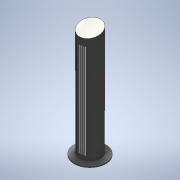
# Autodesk Inventor part: fan
Saved by Autodesk Inventor 2022 (Build 260153000, 153)
## iProperties
Created: 2023-01-12
Part Number: fan
Material: Generic
Document SubType Name: Modeling
Designer: mihir
Density: 1 g/cm^3
Appearance: Default
Author: mihir
Autodesk Inventor part; units mm, degrees
ref_plane "XY Plane" through (0, 0, 0) normal (0, 0, 1) x (1, 0, 0)
sketch "Sketch1" plane through (0, 0, 0) normal (0, 1, 0) x (-1, 0, 0)
  circle A0 centre (0, 0) radius 15
  dimension "d0" = 30
  constraints: 1 centre point, 1 coincident
  measures "d0" diameter of A0
ref_plane "Work Plane1" through (0, 1, 0) normal (0, 1, 0) x (-1, 0, 0)
sketch "Sketch2" plane through (0, 1, 0) normal (0, 1, 0) x (-1, 0, 0)
  circle A0 centre (0, 0) radius 15
  dimension "d2" = 30
  constraints: 1 centre point, 1 coincident
  measures "d2" diameter of A0
ref_plane "Work Plane2" through (0, 2, 0) normal (0, 1, 0) x (-1, 0, 0)
sketch "Sketch4" plane through (0, 2, 0) normal (0, 1, 0) x (-1, 0, 0)
  circle A0 centre (0, 0) radius 10
  dimension "d11" = 20
  constraints: 1 centre point, 1 coincident
  measures "d11" diameter of A0
loft "Loft2" add profiles "Sketch1", "Sketch2"
loft "Loft3" add profiles "Sketch4" section 1 edges at (15, 1, 0)
extrude "Extrusion1" add sketch "Sketch4" along normal blind 100
sketch "Sketch5" plane through (0, 0, 0) normal (0, 0, 1) x (1, 0, 0)
  line L0 (10, 102) -> (-10, 102) projected
  line L1 (-10, 102) -> (10, 102)
  line L2 (10, 102) -> (10, 107)
  line L3 (-10, 102) -> (-10, 102.5)
  line L4 (-10, 102.5) -> (10, 107)
  point P0 (0, 0)
  dimension "d22" = 5
  dimension "d23" = 0.5
  constraints: 8 end point, 1 collinear, 1 perpendicular, 1 vertical
  measures "d22" distance of L0.start L2.end
  measures "d23" distance of L0.end L3.end
extrude "Extrusion2" add sketch "Sketch5" along normal mid plane 20
fillet "Fillet1" radius 10 4 edges at (10, 104.5, 10) (10, 104.5, -10) (-10, 102.25, 10) (-10, 102.25, -10)
ref_plane "Work Plane3" through (-10, 0, 0) normal (1, 0, 0) x (0, 1, 0)
sketch "Sketch6" plane through (-10, 0, 0) normal (1, 0, 0) x (0, 1, 0)
  line L0 (96, -5) -> (6, -5)
  line L1 (6, -5) -> (6, 5)
  line L2 (6, 5) -> (96, 5)
  line L3 (96, 5) -> (96, -5)
  line L4 (0, -15) -> (0, 15) projected
  line L5 (0, -15) -> (1, -15)
  line L6 (0, -15) -> (1, -15) projected
  line L7 (1, 15) -> (1, -15) projected
  line L8 (96, -4) -> (6, -4)
  line L9 (6, -3.5) -> (96, -3.5)
  line L10 (96, -2.5) -> (6, -2.5)
  line L11 (6, -2) -> (96, -2)
  line L12 (96, -1) -> (6, -1)
  line L13 (6, -1) -> (96, -1)
  line L14 (96, -0.5) -> (6, -0.5)
  line L15 (6, 0.5) -> (96, 0.5)
  line L16 (96, 1) -> (6, 1)
  line L17 (96, 2) -> (6, 2)
  line L18 (96, 5) -> (6, 5)
  line L19 (96, 2.5) -> (6, 2.5)
  line L20 (2, 10) -> (104.75, 10) projected
  line L21 (6, 3.5) -> (96, 3.5)
  line L22 (96, 4) -> (6, 4)
  line L23 (6, 4) -> (96, 4)
  point P0 (0, 0)
  point P1 (6, 2.5)
  point P2 (6, 1)
  dimension "d28" = 90
  dimension "d29" = 10
  dimension "d30" = 10
  dimension "d31" = 5
  dimension "d34" = 1
  dimension "d35" = 0.5
  dimension "d36" = 1
  dimension "d37" = 0.5
  dimension "d38" = 1
  dimension "d39" = 0.5
  dimension "d40" = 1
  dimension "d41" = 0.5
  dimension "d42" = 1
  dimension "d43" = 0.5
  dimension "d44" = 1
  dimension "d45" = 1
  dimension "d46" = 0.5
  constraints: 36 end point, 15 horizontal, 2 parallel, 1 collinear, 1 point on line, 29 other
  measures "d28" distance of L2.start L2.end
  measures "d29" distance of L0.end L2.start
  measures "d30" distance between parallel lines of L5 L0
  measures "d34" distance between parallel lines of L0 L8
  measures "d35" distance between parallel lines of L8 L9
  measures "d36" distance between parallel lines of L10 L9
  measures "d37" distance between parallel lines of L10 L11
  measures "d38" distance between parallel lines of L11 L12
  measures "d39" distance between parallel lines of L14 L12
  measures "d40" distance between parallel lines of L14 L15
  measures "d41" distance between parallel lines of L15 L16
  measures "d42" distance between parallel lines of L17 L16
  measures "d43" distance between parallel lines of L17 L19
  measures "d44" distance between parallel lines of L19 L21
  measures "d45" distance between parallel lines of L2 L23
  measures "d46" distance between parallel lines of L21 L22
extrude "Extrusion3" cut sketch "Sketch6" along normal blind 5 contours L0 L1 L8 L3 | L9 L1 L10 L3 | L11 L1 L12 L3 | L14 L1 L15 L3 | L16 L1 L17 L3 | L19 L1 L21 L3 | L22 L1 L2 L3
body "Solid2"
